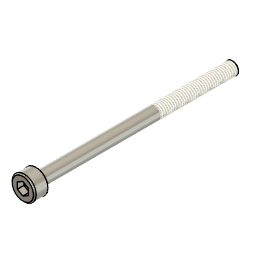
ensamble1_ (Autodesk Fusion 360 archive; units mm, degrees)
design "Tornillo brochado de cabeza hueca hexagonal ASME B18.3.1M - M3x0.5 x 45 Acero grado 2 Normal"
description: Tornillo brochado de cabeza hueca hexagonal ASME B18.3.1M - M3x0.5 x 45
part number: BSHCS ASME B18.3.1M - M3x0.5 x 45 Acero grado 2 Normal
Autodesk Fusion 360 part; units mm, degrees
sketch "Sketch1" plane through (0, 0, 0) normal (0, 1, 0) x (1, 0, 0)
  line L0 (-1.5, 0) -> (-1.5, 45)
  line L1 (-1.5, 45) -> (0, 45)
  line L2 (0, 45) -> (0, -3)
  line L3 (-1.5, 0) -> (-2.75, 0)
  line L4 (-2.75, 0) -> (-2.75, -3)
  line L5 (-2.75, -3) -> (0, -3)
  dimension "d101" = 45
  dimension "d102" = 3
  dimension "d109" = 5.5
  dimension "d110" = 3
  constraint perpendicular L0 L1
  constraint collinear origin L1.end L2.end
  constraint perpendicular L0 L3
  constraint coincident origin L3
  constraint vertical L2
  constraint coincident L2 L5.end
  constraint perpendicular L2 L5
  measures "d101" distance of origin L1
  measures "d102" distance of L3.end L5
revolve "Revolve1" add sketch "Sketch1" angle 360 about axis through (0, 0, -45) along (0, 0, 1)
ref_plane "WorkPlane1" through (0, 0, 3) normal (0, 0, 1) x (1, 0, 0)
sketch "Sketch6" plane through (0, 0, 3) normal (0, 0, 1) x (1, 0, 0)
  line L0 (0, -1.4434) -> (1.25, -0.7217)
  line L1 (1.25, -0.7217) -> (1.25, 0.7217)
  line L2 (1.25, 0.7217) -> (0, 1.4434)
  line L3 (0, 1.4434) -> (-1.25, 0.7217)
  line L4 (-1.25, 0.7217) -> (-1.25, -0.7217)
  line L5 (-1.25, -0.7217) -> (0, -1.4434)
  dimension "d111" = 2.5
  constraint vertical L1
  measures "d111" distance of L1 L4
extrude "Extrude1" cut sketch "Sketch6" against normal blind 1.5
extrude "Extrude2" cut 1 faces at (0, -0.4811, 1.5) along direction (0, 0, -1) blind 1.5 draft -85
thread "Thread3" "ANSI Metric M Profile 3.0 M3x0.5 M3x0.5 4g6g" major diameter 2.927 minor diameter 2.369 pitch 0.5 angle 60 resizes the face on face at (-1.4981, 0.0748, -30) from (0, 0, -27) to (0, 0, -45)
fillet "Fillet4" radius 0.3 1 edges at (-2.5639, 0.9944, 3)
sketch "Sketch7" plane through (0, 0, 0) normal (0, 1, 0) x (1, 0, 0)
  line L0 (-1.53, 45) -> (-1.53, 44.6933)
  line L1 (-1.53, 44.6933) -> (-1.1933, 45)
  line L2 (0, 45) -> (0, -3)
  line L3 (-1.53, 45) -> (0, 45)
  dimension "d104" = 1.1933
  dimension "d105" = 1.53
  dimension "d106" = 0.3067
  constraint coincident L2.start L3.end
  constraint perpendicular L2 L3
  constraint coincident L1.end L3
  constraint perpendicular L0 L3
  measures "d104" distance of L1.end L2
  measures "d105" distance of L0 L2.start
  measures "d106" distance of L0.end L3
revolve "Revolve3" cut sketch "Sketch7" angle 360 about axis through (0, 0, 1.75) along (0, 0, 1)
equation "adsk_nomlen = 45.00 mm"
equation "adsk_headh = 3.00 mm"
equation "adsk_headdia = 5.50 mm"
equation "adsk_nomdia = 3.00 mm"
equation "adsk_philwidth = 2.50 mm"
equation "d31 = -adsk_phildepth"
equation "adsk_phildepth = 1.50 mm"
equation "d71 = adsk_headh"
equation "d76 = -adsk_phildepth"
equation "adsk_thrlen = 18.00 mm"
equation "d86 = adsk_nomdia * 0.1"
equation "adsk_startlen = 0.306725 mm"
equation "adsk_endpointdia = 2.38655 mm"
equation "d101 = adsk_nomlen"
equation "d102 = adsk_headh"
equation "d104 = adsk_endpointdia / 2"
equation "d105 = adsk_nomdia * 0.51"
equation "d106 = adsk_startlen"
equation "d108 = min(adsk_thrlen; adsk_nomlen - 0.001 mm)"
equation "d109 = adsk_headdia"
equation "d110 = adsk_nomdia"
equation "d111 = adsk_philwidth"

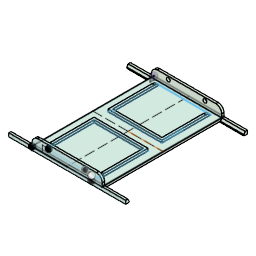
design "baseInferior"
Autodesk Fusion 360 part; units mm, degrees
sketch "Boceto1" plane through (0, 0, 0) normal (0, 0, 1) x (1, 0, 0)
  line L0 (0, 0) -> (0, -104)
  line L1 (0, 0) -> (60, 0)
  line L2 (60, 0) -> (60, -104)
  line L3 (0, -104) -> (60, -104)
  line L4 (60, 0) -> (60, -2)
  line L5 (60, -2) -> (0, -2)
  line L6 (60, -104) -> (60, -102)
  line L7 (60, -102) -> (0, -102)
  line L8 (0, -104) -> (30, -104)
  line L9 (30, -52) -> (60, -52) construction
  line L10 (0, -52) -> (60, -52) construction
  line L11 (30, -2) -> (51, -2) construction
  line L12 (51, -4.5) -> (51, -42)
  line L13 (9, -42) -> (9, -4.5)
  line L14 (30, -102) -> (51, -102) construction
  line L15 (51, -99.5) -> (51, -62)
  line L16 (9, -62) -> (9, -99.5)
  line L17 (53, -44) -> (53, -4.5)
  line L18 (7, -44) -> (7, -4.5)
  line L19 (53, -60) -> (53, -99.5)
  line L20 (7, -60) -> (7, -99.5)
  line L21 (7, -4.5) -> (53, -4.5)
  line L22 (30, -2) -> (30, 0) construction
  line L23 (7, -4.5) -> (53, -4.5)
  line L24 (7, -99.5) -> (53, -99.5)
  line L25 (30, -104) -> (30, -102) construction
  line L26 (53, -60) -> (53, -58)
  line L27 (53, -58) -> (7, -58)
  line L28 (7, -58) -> (7, -60)
  line L29 (9, -62) -> (9, -60)
  line L30 (9, -60) -> (51, -60)
  line L31 (51, -60) -> (51, -62)
  line L32 (30, -99.5) -> (30, -44) construction
  line L33 (30, -42) -> (30, -4.5) construction
  line L34 (7, -44) -> (7, -46)
  line L35 (7, -46) -> (53, -46)
  line L36 (53, -46) -> (53, -28.3409)
  line L37 (9, -42) -> (9, -44)
  line L38 (9, -44) -> (51, -44)
  line L39 (51, -44) -> (51, -26.5441)
  dimension "d1" = 104
  dimension "d2" = 60
  dimension "d3" = 104
  dimension "d4" = 2
  dimension "d5" = 2
  dimension "d14" = 21
  dimension "d15" = 40
  dimension "d16" = 42
  dimension "d17" = 21
  dimension "d18" = 40
  dimension "d19" = 42
  dimension "d26" = 46
  dimension "d64" = 2
  dimension "d65" = 2
  dimension "d66" = 2
  dimension "d67" = 2
  constraint coincident L0.start L1.start
  constraint vertical L0
  constraint perpendicular L0 L1
  constraint perpendicular L1 L2
  constraint perpendicular L1 L4
  constraint coincident L0 L5.end
  constraint perpendicular L0 L5
  constraint perpendicular L3 L6
  constraint coincident L0 L7.end
  constraint perpendicular L0 L7
  constraint midpoint L3 L8.end
  constraint midpoint L1 L22.end
  constraint midpoint L2 L9.end
  constraint midpoint L0 L10.start
  constraint midpoint L5 L11.start
  constraint perpendicular L11 L25
  constraint perpendicular L11 L12
  constraint perpendicular L5 L13
  constraint midpoint L7 L14.start
  constraint perpendicular L14 L25
  constraint perpendicular L14 L15
  constraint perpendicular L7 L16
  constraint perpendicular L5 L17
  constraint perpendicular L5 L18
  constraint perpendicular L7 L19
  constraint perpendicular L7 L20
  constraint perpendicular L17 L21
  constraint coincident L21 L13.end
  constraint coincident L21 L33.end
  constraint collinear L22 L25
  constraint coincident L9.start L25
  constraint coincident L21 L12.start
  constraint perpendicular L19 L24
  constraint coincident L24 L15.start
  constraint coincident L24 L32.start
  constraint collinear L25 L32
  constraint coincident L24 L16.end
  constraint perpendicular L20 L27
  constraint perpendicular L27 L28
  constraint perpendicular L10 L29
  constraint perpendicular L15 L30
  constraint perpendicular L30 L31
  constraint coincident L33.start L32
  constraint collinear L32 L33
  constraint parallel L18 L34
  constraint perpendicular L17 L35
  constraint coincident L17 L36.end
  constraint perpendicular L35 L36
  constraint parallel L13 L37
  constraint perpendicular L12 L38
  constraint coincident L12 L39.end
  constraint perpendicular L38 L39
  measures "d1" distance of L0.start L0.end
  measures "d2" distance of L0.start L1.end
  measures "d3" distance of L1.end L2.end
  measures "d4" distance of L1.end L4.end
  measures "d5" distance of L2.end L6.end
  measures "d14" distance of L11.start L11.end
  measures "d15" distance of L11.end L12.end
  measures "d16" distance of L12.end L13.start
  measures "d17" distance of L14.start L14.end
  measures "d18" distance of L14.end L15.end
  measures "d19" distance of L15.end L16.start
  measures "d26" distance of L19.start L20.start
  measures "d64" distance of L19.start L26.end
  measures "d65" distance of L16.start L29.end
  measures "d66" distance of L18.start L34.end
  measures "d67" distance of L13.start L37.end
extrude "Extruir1" add sketch "Boceto1" against normal blind 2 contours L0 L1 L2 L4 L5 | L0 L2 L5 L7 | L0 L2 L3 L6 L7 L8 | L12 L13 L17 L18 L21 L23 L34 L35 L36 L37 L38 L39 | L12 L13 L21 L23 L37 L38 L39 | L15 L16 L24 L29 L30 L31 | L15 L16 L19 L20 L24 L26 L27 L28 L29 L30 L31
extrude "Extruir2" add sketch "Boceto1" along normal blind 8 contours L0 L1 L2 L4 L5 | L0 L2 L3 L6 L7 L8
fillet "Empalme1" radius 5 1 edges at (0, -103, 8)
fillet "Empalme2" radius 5 3 edges at (60, -103, 8) (0, -1, 8) (60, -1, 8)
extrude "Extruir3" add sketch "Boceto1" along normal blind 2 contours L15 L16 L19 L20 L24 L26 L27 L28 L29 L30 L31
extrude "Extruir4" add sketch "Boceto1" along normal blind 2 contours L12 L13 L17 L18 L21 L23 L34 L35 L36 L37 L38 L39
fillet "Empalme4" radius 5 1 edges at (8, -99.5, 2)
fillet "Empalme5" radius 5 1 edges at (52, -99.5, 2)
fillet "Empalme6" radius 5 2 edges at (8, -4.5, 2) (52, -4.5, 2)
sketch "Boceto2" plane through (0, 0, 0) normal (1, 0, 0) x (0, 1, 0)
  line L0 (0, 0) -> (0, -3)
  line L1 (0, -3) -> (-3, -3)
  line L2 (-3, -3) -> (-3, -2)
  line L3 (0, 0) -> (-2, 0)
  line L4 (-2, 0) -> (-3, -2)
  line L5 (0, 0) -> (-104, 0) construction
  line L6 (-104, 0) -> (-102, 0)
  line L7 (-104, 0) -> (-104, -3)
  line L8 (-104, -3) -> (-101, -3)
  line L9 (-101, -3) -> (-101, -2)
  line L10 (-101, -2) -> (-102, 0)
  dimension "d42" = 3
  dimension "d43" = 3
  dimension "d44" = 1
  dimension "d45" = 2
  dimension "d46" = 104
  dimension "d47" = 2
  dimension "d48" = 3
  dimension "d49" = 3
  dimension "d50" = 1
  constraint coincident L0.start L3.start
  constraint vertical L0
  constraint perpendicular L0 L1
  constraint perpendicular L1 L2
  constraint perpendicular L2 L3
  constraint perpendicular L0 L5
  constraint parallel L5 L6
  constraint perpendicular L6 L7
  constraint perpendicular L7 L8
  constraint perpendicular L8 L9
  measures "d42" distance of L0.start L0.end
  measures "d43" distance of L0.end L1.end
  measures "d44" distance of L1.end L2.end
  measures "d45" distance of L0.start L3.end
  measures "d46" distance of L0.start L5.end
  measures "d47" distance of L5.end L6.end
  measures "d48" distance of L5.end L7.end
  measures "d49" distance of L7.end L8.end
  measures "d50" distance of L8.end L9.end
extrude "Extruir5" add sketch "Boceto2" along normal blind 80 and the other way blind 20
sketch "Boceto3" plane through (0, -104, 0) normal (0, -1, 0) x (1, 0, 0)
  line L0 (60, 0) -> (60, 3)
  arc A0 (60, 3) -> (55, 8) centre (55, 3) ccw
  line L1 (55, 8) -> (5, 8)
  arc A1 (5, 8) -> (0, 3) centre (5, 3) ccw
  line L2 (0, 3) -> (0, 0)
  line L3 (0, 0) -> (-20, 0)
  line L4 (-20, 0) -> (-20, -3)
  line L5 (-20, -3) -> (80, -3)
  line L6 (80, -3) -> (80, 0)
  line L7 (80, 0) -> (60, 0)
  line L8 (0, 0) -> (30, 0) construction
  line L9 (30, 0) -> (51, 0) construction
  line L10 (51, 3.9) -> (51, 5.4) construction
  line L11 (30, 0) -> (9, 0) construction
  line L12 (9, 0) -> (9, 5.4) construction
  line L13 (9, 5.4) -> (14.4, 5.4) construction
  line L14 (51, 5.4) -> (45.6, 5.4) construction
  circle A2 centre (45.6, 5.4) radius 1.6
  circle A3 centre (14.4, 5.4) radius 1.6
  dimension "d55" = 30
  dimension "d56" = 21
  dimension "d57" = 5.4
  dimension "d59" = 21
  dimension "d60" = 5.4
  dimension "d68" = 5.4
  dimension "d69" = 5.4
  dimension "d70" = 3.2
  dimension "d71" = 3.2
  constraint coincident L2.end L3.start
  constraint perpendicular L0 L8
  constraint parallel L8 L9
  constraint perpendicular L1 L10
  constraint parallel L8 L11
  constraint perpendicular L8 L12
  constraint perpendicular L12 L13
  constraint perpendicular L10 L14
  constraint coincident L14.end A2.centre
  constraint coincident L13.end A3.centre
  measures "d55" distance of L2.end L8.end
  measures "d56" distance of L8.end L9.end
  measures "d57" distance of L9.end L10.end
  measures "d59" distance of L8.end L11.end
  measures "d60" distance of L11.end L12.end
  measures "d68" distance of L12.end L13.end
  measures "d69" distance of L10.end L14.end
  measures "d70" diameter of A2
  measures "d71" diameter of A3
extrude "Extruir7" cut sketch "Boceto3" along normal mid plane 2000 contours A2 | A3

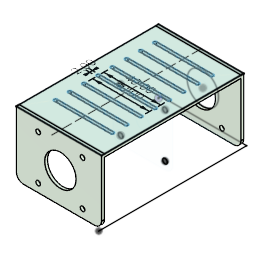
design "baseSuperior"
Autodesk Fusion 360 part; units mm, degrees
sketch "Boceto6" plane through (0, 0, 0) normal (0, 0, 1) x (1, 0, 0)
  line L0 (0, 0) -> (60, 0)
  line L1 (60, 0) -> (60, -100)
  line L2 (0, 0) -> (0, -100)
  line L3 (0, -100) -> (60, -100)
  line L4 (0, 0) -> (60, 0)
  line L5 (60, 0) -> (60, -2)
  line L6 (60, -2) -> (0, -2)
  line L7 (0, -100) -> (0, -98.9254)
  line L8 (0, -100) -> (0, -98)
  line L9 (0, -98) -> (60, -98)
  line L10 (30, 0) -> (30, -104.8793) construction
  line L11 (50, -51.4397) -> (10, -51.4397) construction
  line L12 (10, -53.4397) -> (50, -53.4397) construction
  line L13 (10, -51.4397) -> (50, -51.4397)
  line L14 (50, -53.4397) -> (10, -53.4397)
  arc A0 (10, -51.4397) -> (10, -53.4397) centre (10, -52.4397) ccw
  arc A1 (50, -53.4397) -> (50, -51.4397) centre (50, -52.4397) ccw
  line L15 (10, -83.4397) -> (50, -83.4397) construction
  arc A2 (10, -81.4397) -> (10, -83.4397) centre (10, -82.4397) ccw
  arc A3 (50, -83.4397) -> (50, -81.4397) centre (50, -82.4397) ccw
  line L16 (50, -81.4397) -> (10, -81.4397) construction
  line L17 (10, -81.4397) -> (50, -81.4397)
  line L18 (50, -83.4397) -> (10, -83.4397)
  line L19 (10, -73.4397) -> (50, -73.4397) construction
  arc A4 (10, -71.4397) -> (10, -73.4397) centre (10, -72.4397) ccw
  arc A5 (50, -73.4397) -> (50, -71.4397) centre (50, -72.4397) ccw
  line L20 (50, -71.4397) -> (10, -71.4397) construction
  line L21 (10, -71.4397) -> (50, -71.4397)
  line L22 (50, -73.4397) -> (10, -73.4397)
  line L23 (10, -63.4397) -> (50, -63.4397) construction
  arc A6 (10, -61.4397) -> (10, -63.4397) centre (10, -62.4397) ccw
  arc A7 (50, -63.4397) -> (50, -61.4397) centre (50, -62.4397) ccw
  line L24 (50, -61.4397) -> (10, -61.4397) construction
  line L25 (10, -61.4397) -> (50, -61.4397)
  line L26 (50, -63.4397) -> (10, -63.4397)
  line L27 (10, -43.4397) -> (50, -43.4397) construction
  arc A8 (10, -41.4397) -> (10, -43.4397) centre (10, -42.4397) ccw
  arc A9 (50, -43.4397) -> (50, -41.4397) centre (50, -42.4397) ccw
  line L28 (50, -41.4397) -> (10, -41.4397) construction
  line L29 (10, -41.4397) -> (50, -41.4397)
  line L30 (50, -43.4397) -> (10, -43.4397)
  line L31 (10, -33.4397) -> (50, -33.4397) construction
  arc A10 (10, -31.4397) -> (10, -33.4397) centre (10, -32.4397) ccw
  arc A11 (50, -33.4397) -> (50, -31.4397) centre (50, -32.4397) ccw
  line L32 (50, -31.4397) -> (10, -31.4397) construction
  line L33 (10, -31.4397) -> (50, -31.4397)
  line L34 (50, -33.4397) -> (10, -33.4397)
  line L35 (10, -23.4397) -> (50, -23.4397) construction
  arc A12 (10, -21.4397) -> (10, -23.4397) centre (10, -22.4397) ccw
  arc A13 (50, -23.4397) -> (50, -21.4397) centre (50, -22.4397) ccw
  line L36 (50, -21.4397) -> (10, -21.4397) construction
  line L37 (10, -21.4397) -> (50, -21.4397)
  line L38 (50, -23.4397) -> (10, -23.4397)
  line L39 (10, -13.4397) -> (50, -13.4397) construction
  arc A14 (10, -11.4397) -> (10, -13.4397) centre (10, -12.4397) ccw
  arc A15 (50, -13.4397) -> (50, -11.4397) centre (50, -12.4397) ccw
  line L40 (50, -11.4397) -> (10, -11.4397) construction
  line L41 (10, -11.4397) -> (50, -11.4397)
  line L42 (50, -13.4397) -> (10, -13.4397)
  dimension "d3" = 60
  dimension "d4" = 100
  dimension "d7" = 2
  dimension "d8" = 2
  dimension "d48" = 1
  dimension "d49" = 40
  dimension "d50" = 2
  dimension "d51" = 40
  dimension "d52" = 2
  dimension "d53" = 2
  dimension "d56" = 0
  dimension "d57" = 40
  constraint coincident L0.start L2.start
  constraint horizontal L0
  constraint perpendicular L0 L1
  constraint perpendicular L0 L2
  constraint perpendicular L1 L3
  constraint vertical L5
  constraint coincident L2 L6.end
  constraint perpendicular L2 L6
  constraint coincident L2 L7.end
  constraint perpendicular L3 L8
  constraint coincident L1 L9.end
  constraint perpendicular L1 L9
  constraint midpoint L0 L10.start
  constraint perpendicular L3 L10
  constraint perpendicular L10 L11
  measures "d3" distance of L0.start L0.end
  measures "d4" distance of L0.end L1.end
  measures "d7" distance of L0.end L5.end
  measures "d8" distance of L2.end L8.end
  measures "d48" distance of L11.start A1.centre
  measures "d49" distance of L11.start L11.end
  measures "d50" distance of L11.end L12.start
  measures "d51" distance of L12.start L12.end
  measures "d52" diameter of A1
  measures "d53" diameter of A0
extrude "Extruir1" add sketch "Boceto6" against normal blind 2 contours L0 L1 L2 L4 L5 L6 | L1 L2 L6 L9 | L1 L2 L3 L7 L8 L9 | L13 L14 A0 A1 | A2 A3 L17 L18 | A4 A5 L21 L22 | A6 A7 L25 L26 | A8 A9 L29 L30 | A10 A11 L33 L34 | A12 A13 L37 L38 | A14 A15 L41 L42
extrude "Extruir2" add sketch "Boceto6" against normal blind 45 contours L0 L1 L2 L4 L5 L6
extrude "Extruir3" add sketch "Boceto6" against normal blind 45 contours L1 L2 L3 L7 L8 L9
fillet "Empalme1" radius 5 1 edges at (60, -99, -45)
fillet "Empalme2" radius 5 2 edges at (60, -1, -45) (0, -99, -45)
fillet "Empalme3" radius 5 1 edges at (0, -1, -45)
sketch "Boceto7" plane through (0, 0, -45) normal (0, 0, -1) x (1, 0, 0)
  line L0 (5, 2) -> (5, 0)
  line L1 (5, 0) -> (55, 0)
  line L2 (55, 0) -> (55, 2)
  line L3 (55, 2) -> (5, 2)
  line L4 (0, 0) -> (0, -2)
  line L5 (0, -2) -> (60, -2)
  line L6 (60, -2) -> (60, 102)
  dimension "d31" = 2
  dimension "d32" = 60
  dimension "d33" = 104
  constraint coincident L4.start origin
  constraint vertical L4
  constraint perpendicular L4 L5
  constraint perpendicular L5 L6
  measures "d31" distance of L4.start L4.end
  measures "d32" distance of L4.end L5.end
  measures "d33" distance of L5.end L6.end
sketch "Boceto8" plane through (0, -42, 0) normal (0, -1, 0) x (1, 0, 0)
  arc A0 (10, -39.5) -> (15, -44.5) centre (15, -39.5) ccw
  line L0 (15, -44.5) -> (47, -44.5)
  arc A1 (47, -44.5) -> (52, -39.5) centre (47, -39.5) ccw
  line L1 (52, -39.5) -> (52, -7.5)
  arc A2 (52, -7.5) -> (47, -2.5) centre (47, -7.5) ccw
  line L2 (47, -2.5) -> (15, -2.5)
  arc A3 (15, -2.5) -> (10, -7.5) centre (15, -7.5) ccw
  line L3 (10, -7.5) -> (10, -15.5)
  line L4 (10, -15.5) -> (6, -15.5)
  line L5 (6, -15.5) -> (6, -31.5)
  line L6 (6, -31.5) -> (10, -31.5)
  line L7 (10, -31.5) -> (10, -39.5)
  circle A4 centre (46.6, -7.9) radius 3
  circle A5 centre (46.6, -39.1) radius 3
  circle A6 centre (15.4, -7.9) radius 3
  circle A7 centre (15.4, -39.1) radius 3
  circle A8 centre (31, -23.5) radius 4.6
  circle A9 centre (15.4, -7.9) radius 1.6
  circle A10 centre (46.6, -7.9) radius 1.6
  circle A11 centre (46.6, -39.1) radius 1.6
  circle A12 centre (15.4, -39.1) radius 1.6
  dimension "d34" = 3.2
  dimension "d35" = 3.2
  dimension "d36" = 3.2
  dimension "d37" = 3.2
  constraint concentric A6 A9
  constraint concentric A4 A10
  constraint concentric A5 A11
  constraint concentric A7 A12
  measures "d34" diameter of A9
  measures "d35" diameter of A10
  measures "d36" diameter of A11
  measures "d37" diameter of A12
extrude "Extruir4" cut sketch "Boceto8" along normal blind 120 and the other way blind 100 contours A9 | A10 | A11 | A12
sketch "Boceto9" plane through (0, 0.2, 0) normal (0, 1, 0) x (-1, 0, 0)
  circle A0 centre (-31, -23.5) radius 11
  circle A1 centre (-31, -23.5) radius 4.6
  circle A2 centre (-31, -23.5) radius 11
  dimension "d42" = 22
  constraint concentric A0 A2
  measures "d42" diameter of A2
extrude "Extruir5" cut sketch "Boceto9" along normal blind 0 and the other way blind 200 contours A0 A2 | A1
extrude "Extruir6" cut sketch "Boceto6" along normal mid plane 20 contours L13 L14 A0 A1 | A2 A3 L17 L18 | A4 A5 L21 L22 | A6 A7 L25 L26 | A8 A9 L29 L30 | A10 A11 L33 L34 | A12 A13 L37 L38 | A14 A15 L41 L42

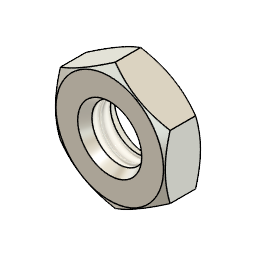
design "Tuerca fina hexagonal DIN 439-2 - M3.5 x 0.6 Acero 6 Normal"
description: Tuerca fina hexagonal DIN 439-2 - M3.5 x 0.6
part number: DIN 439-2 - M3.5 x 0.6 Acero 6 Normal
Autodesk Fusion 360 part; units mm, degrees
sketch "Sketch1" plane through (0, 0, 0) normal (0, 1, 0) x (1, 0, 0)
  line L0 (0, 0) -> (0, -2)
  line L1 (-1.75, 0) -> (-2.94, 0)
  line L2 (-2.94, 0) -> (-3.465, -0.3031)
  line L3 (-3.465, -0.3031) -> (-3.465, -1.6969)
  line L4 (-3.465, -1.6969) -> (-2.94, -2)
  line L5 (-2.94, -2) -> (-1.75, -2)
  line L6 (-1.75, -2) -> (-1.75, 0)
  dimension "d121" = 3.5
  dimension "d122" = 30
  dimension "d123" = 30
  dimension "d128" = 6.93
  dimension "d172" = 5.88
  dimension "d179" = 2
  constraint vertical L0
  constraint coincident L0 L0.end
  constraint coincident origin L0
  constraint horizontal L1
  constraint coincident L0.start L1
  constraint coincident L0.start origin
  constraint coincident L0.end L5
  constraint vertical L1.end L4.end
  measures "d122" angle of L1 L2
  measures "d123" angle of L4 L5
  measures "d179" distance of L1 L5
revolve "Revolve1" add sketch "Sketch1" angle 360 about axis through (0, 0, 0) along (0, 0, 1)
sketch "Sketch8" plane through (0, 0, 2) normal (0, 0, 1) x (1, 0, 0)
  line L0 (-3, -1.7338) -> (-3, 1.7338)
  circle A0 centre (0, 0) radius 1.75
  circle A1 centre (0, 0) radius 3.465
  dimension "d114" = 3
  constraint coincident L0.end A1
  constraint coincident L0.start A1
  constraint vertical L0
  measures "d114" distance of A0.centre L0
extrude "Extrude5" cut sketch "Sketch8" against normal blind 2 contours L0 A1 picked at (-3.075, 0.4223)
pattern_circular "C-Pattern2" count 6 over 360 about axis through (0, 0, 1.75) along (0, 0, 1) of "Extrude5"
thread "Thread3" "ISO Metric profile 3.5 M3.5x0.6 M3.5x0.6 6H" major diameter 3.5995 minor diameter 2.93 pitch 0.6 angle 60 resizes the face on face at (-1.7413, 0.1742, 1.3333)
sketch "Sketch12" plane through (0, 0, 0) normal (0, 1, 0) x (1, 0, 0)
  line L0 (-1.75, 0) -> (0, 0)
  line L1 (-1.1726, -1) -> (-1.75, 0)
  line L2 (-1.75, -2) -> (0, -2)
  line L3 (-1.1726, -1) -> (-1.75, -2)
  line L4 (0, 0) -> (0, -2)
  dimension "d169" = 60
  dimension "d177" = 1.75
  dimension "d178" = 60
  constraint horizontal L0
  constraint coincident L1.start L3.start
  constraint vertical L0.start L2.start
  constraint coincident L2.end L4.end
  constraint coincident L0.end L4.start
  constraint perpendicular L2 L4
  measures "d169" angle of L2 L3
  measures "d177" distance of L0.start L4
  measures "d178" angle of L0 L1
revolve "Revolve3" cut sketch "Sketch12" angle 360 about axis through (0, 0, 1.75) along (0, 0, 1)
equation "adsk_nheig = 2.00 mm"
equation "adsk_maxdia = 6.93 mm"
equation "adsk_nomdia = 3.50 mm"
equation "d89 = -adsk_nheig"
equation "adsk_waflat = 6.00 mm"
equation "d114 = adsk_waflat / 2"
equation "adsk_chamang1 = 30.00 deg"
equation "adsk_chamang2 = 30.00 deg"
equation "d121 = adsk_nomdia"
equation "d122 = adsk_chamang1"
equation "d123 = adsk_chamang2"
equation "d128 = adsk_maxdia"
equation "d163 = adsk_nheig"
equation "adsk_beardia = 5.88 mm"
equation "d172 = adsk_beardia"
equation "d177 = adsk_nomdia * 0.5"
equation "d179 = adsk_nheig"
